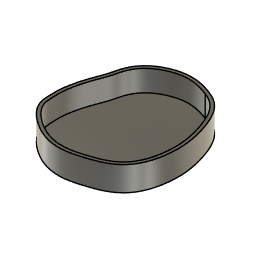
arm cover v3 (Autodesk Fusion 360 design; units mm, degrees)
Autodesk Fusion 360 part; units mm, degrees
sketch "Sketch1" plane through (0, 0, 0) normal (0, 0, 1) x (1, 0, 0)
  spline S0 degree 5 poles (4, 24) (4.2976, 23.8824) (4.8869, 23.6403) (5.7529, 23.2536) (6.872, 22.6708) (8.2119, 21.7595) (9.4914, 20.595) (10.706, 19.1267) (11.8468, 17.347) (12.9002, 15.3034) (13.8506, 13.0778) (14.6827, 10.7718) (15.3841, 8.4902) (15.9477, 6.3241) (16.3742, 4.3363) (16.6747, 2.5415) (16.8679, 0.9163) (16.9746, -0.5863) (17.014, -2.0239) (16.9985, -3.4508) (16.9299, -4.9045) (16.802, -6.407) (16.6033, -7.9648) (16.32, -9.5705) (15.9388, -11.2023) (15.4478, -12.8286) (14.8364, -14.413) (14.0949, -15.9199) (13.215, -17.3192) (12.1891, -18.5923) (11.0125, -19.7312) (9.6846, -20.7375) (8.2112, -21.6215) (6.6057, -22.4017) (4.8902, -23.1029) (3.0899, -23.7487) (1.2285, -24.3557) (-0.677, -24.9264) (-2.6203, -25.4435) (-4.6118, -25.8615) (-6.6717, -26.1171) (-8.8195, -26.1424) (-11.0657, -25.8772) (-13.4017, -25.2823) (-15.7921, -24.3507) (-18.162, -23.1234) (-20.4096, -21.6797) (-22.4258, -20.1182) (-24.1112, -18.5416) (-25.3954, -17.0399) (-26.253, -15.6745) (-26.7254, -14.4599) (-26.9274, -13.354) (-26.9931, -12.2827) (-27.0347, -11.1584) (-27.0876, -9.9025) (-27.1236, -8.4555) (-27.0862, -6.7846) (-26.9165, -4.8906) (-26.5879, -2.8189) (-26.1113, -0.6517) (-25.5211, 1.5133) (-24.867, 3.5786) (-24.2034, 5.467) (-23.5799, 7.1366) (-23.0304, 8.6046) (-22.5693, 9.9353) (-22.1911, 11.2109) (-21.8693, 12.5083) (-21.5539, 13.8703) (-21.1757, 15.2944) (-20.6627, 16.7519) (-19.9522, 18.1989) (-19.0061, 19.5914) (-17.8225, 20.8967) (-16.4248, 22.0905) (-14.8534, 23.154) (-13.1569, 24.0721) (-11.3826, 24.8303) (-9.5686, 25.413) (-7.7444, 25.8067) (-5.9328, 26.004) (-4.1503, 26.0067) (-2.409, 25.8296) (-0.7174, 25.505) (0.919, 25.0735) (2.1813, 24.6712) (3.1011, 24.3461) (3.7024, 24.1176) (4, 24) knots 0 0 0 0 0 0 0.01176471 0.02352941 0.03529412 0.04705882 0.05882353 0.07058824 0.08235294 0.09411765 0.10588235 0.11764706 0.12941176 0.14117647 0.15294118 0.16470588 0.17647059 0.18823529 0.2 0.21176471 0.22352941 0.23529412 0.24705882 0.25882353 0.27058824 0.28235294 0.29411765 0.30588235 0.31764706 0.32941176 0.34117647 0.35294118 0.36470588 0.37647059 0.38823529 0.4 0.41176471 0.42352941 0.43529412 0.44705882 0.45882353 0.47058824 0.48235294 0.49411765 0.50588235 0.51764706 0.52941176 0.54117647 0.55294118 0.56470588 0.57647059 0.58823529 0.6 0.61176471 0.62352941 0.63529412 0.64705882 0.65882353 0.67058824 0.68235294 0.69411765 0.70588235 0.71764706 0.72941176 0.74117647 0.75294118 0.76470588 0.77647059 0.78823529 0.8 0.81176471 0.82352941 0.83529412 0.84705882 0.85882353 0.87058824 0.88235294 0.89411765 0.90588235 0.91764706 0.92941176 0.94117647 0.95294118 0.96470588 0.97647059 0.98823529 1 1 1 1 1 1
  spline S1 degree 3 poles (4.9189, 26.325) (6.4748, 25.71) (8.0541, 24.968) (9.5874, 23.7829) (11.1792, 22.5526) (12.6425, 20.8269) (13.8702, 18.7373) (15.8899, 15.2997) (17.3679, 10.9247) (18.2619, 7.2921) (18.8769, 4.7933) (19.212, 2.6577) (19.3718, 0.7792) (19.5566, -1.3936) (19.5431, -3.2862) (19.3897, -5.3641) (19.2287, -7.5453) (18.8857, -9.9413) (18.1731, -12.396) (17.4873, -14.7578) (16.448, -17.1407) (14.8923, -19.1745) (13.489, -21.0092) (11.657, -22.5189) (9.6061, -23.6634) (7.6112, -24.7767) (5.446, -25.59) (3.2201, -26.3281) (1.1841, -27.0032) (-0.9009, -27.6409) (-3.2065, -28.1024) (-5.3968, -28.5409) (-7.8266, -28.7707) (-10.4262, -28.4313) (-13.0358, -28.0907) (-15.7974, -27.1537) (-18.3867, -25.7846) (-21.1672, -24.3144) (-23.7206, -22.4028) (-25.5919, -20.519) (-27.1445, -18.956) (-28.2367, -17.3891) (-28.8184, -15.8883) (-29.2502, -14.774) (-29.3878, -13.7475) (-29.4511, -12.9035) (-29.5261, -11.9028) (-29.5469, -11.0754) (-29.581, -9.9629) (-29.6197, -8.6986) (-29.6328, -7.0787) (-29.4342, -5.1952) (-29.1656, -2.6483) (-28.485, 0.3227) (-27.6743, 2.9569) (-27.0382, 5.024) (-26.3522, 6.8515) (-25.8115, 8.3076) (-25.2553, 9.8055) (-24.8726, 10.9085) (-24.557, 12.0964) (-24.2827, 13.1287) (-24.0484, 14.2937) (-23.6471, 15.6573) (-23.1884, 17.2158) (-22.4592, 18.9986) (-21.2879, 20.6179) (-19.7332, 22.7673) (-17.4837, 24.5713) (-15.0074, 25.8866) (-11.8886, 27.543) (-8.3863, 28.4728) (-5.0437, 28.482) (-2.733, 28.4883) (-0.5445, 28.0655) (1.4266, 27.5065) (2.6452, 27.1608) (3.7905, 26.771) (4.9189, 26.325) knots 0 0 0 0 0.03405552 0.03405552 0.03405552 0.06941006 0.06941006 0.06941006 0.12757193 0.12757193 0.12757193 0.16757966 0.16757966 0.16757966 0.21385419 0.21385419 0.21385419 0.2624294 0.2624294 0.2624294 0.30916723 0.30916723 0.30916723 0.35132881 0.35132881 0.35132881 0.39233682 0.39233682 0.39233682 0.42984722 0.42984722 0.42984722 0.46548177 0.46548177 0.46548177 0.50125441 0.50125441 0.50125441 0.53966828 0.53966828 0.53966828 0.5715399 0.5715399 0.5715399 0.59520385 0.59520385 0.59520385 0.62325635 0.62325635 0.62325635 0.65513731 0.65513731 0.65513731 0.69824515 0.69824515 0.69824515 0.73207311 0.73207311 0.73207311 0.76687413 0.76687413 0.76687413 0.79711827 0.79711827 0.79711827 0.83168571 0.83168571 0.83168571 0.87756774 0.87756774 0.87756774 0.9353539 0.9353539 0.9353539 0.97530131 0.97530131 0.97530131 1 1 1 1
  spline S2 degree 3 poles (5.4703, 27.72) (6.8981, 27.1557) (8.3804, 26.4768) (9.8776, 25.4307) (11.4843, 24.308) (13.0235, 22.7418) (14.3025, 20.8608) (16.2773, 17.9567) (17.7523, 14.3146) (18.8152, 10.8952) (19.5951, 8.3861) (20.1346, 6.0472) (20.4726, 4.017) (20.9323, 1.2555) (21.0378, -0.9634) (20.9931, -3.1848) (20.9542, -5.1171) (20.7976, -7.1205) (20.4174, -9.3083) (19.9666, -11.9023) (19.1978, -14.7226) (17.8111, -17.3661) (16.7276, -19.4316) (15.2256, -21.3659) (13.3818, -22.9008) (11.3936, -24.5559) (9.0775, -25.7248) (6.7476, -26.6495) (4.623, -27.4927) (2.4871, -28.1832) (0.1987, -28.8187) (-1.8091, -29.3762) (-3.9937, -29.8986) (-6.4754, -30.0538) (-8.8321, -30.2011) (-11.4382, -29.9579) (-14.0433, -29.1906) (-17.9011, -28.0542) (-21.7394, -25.8145) (-24.6953, -23.3621) (-26.5497, -21.8236) (-28.0514, -20.2274) (-29.108, -18.5854) (-29.9068, -17.3441) (-30.4328, -16.0283) (-30.6869, -14.8726) (-30.9062, -13.8755) (-30.9514, -13.0594) (-30.9866, -12.371) (-31.0292, -11.5369) (-31.0593, -10.7896) (-31.0866, -9.7902) (-31.1227, -8.4752) (-31.1206, -6.7466) (-30.8976, -4.7792) (-30.5937, -2.0973) (-29.8694, 0.9581) (-29.0376, 3.6251) (-28.3807, 5.7316) (-27.6846, 7.5697) (-27.1564, 8.995) (-26.6859, 10.2644) (-26.3612, 11.1981) (-26.0933, 12.1625) (-25.8477, 13.0466) (-25.6398, 14.0276) (-25.3126, 15.2666) (-24.9561, 16.6168) (-24.435, 18.2487) (-23.5374, 19.8695) (-22.5637, 21.6277) (-21.1605, 23.2993) (-19.52, 24.67) (-17.1742, 26.6301) (-14.4032, 28.0625) (-11.5186, 28.9633) (-8.9709, 29.7589) (-6.2911, 30.0928) (-3.7638, 29.9464) (-1.5974, 29.821) (0.4037, 29.3745) (2.2064, 28.8423) (3.3403, 28.5075) (4.405, 28.141) (5.4703, 27.72) knots 0 0 0 0 0.02986894 0.02986894 0.02986894 0.0619222 0.0619222 0.0619222 0.11141063 0.11141063 0.11141063 0.14772296 0.14772296 0.14772296 0.19711607 0.19711607 0.19711607 0.24008138 0.24008138 0.24008138 0.29102442 0.29102442 0.29102442 0.33083009 0.33083009 0.33083009 0.37375435 0.37375435 0.37375435 0.4128947 0.4128947 0.4128947 0.44723405 0.44723405 0.44723405 0.47984322 0.47984322 0.47984322 0.52813476 0.52813476 0.52813476 0.55842912 0.55842912 0.55842912 0.58133166 0.58133166 0.58133166 0.60109042 0.60109042 0.60109042 0.62502929 0.62502929 0.62502929 0.65652392 0.65652392 0.65652392 0.69945843 0.69945843 0.69945843 0.73337113 0.73337113 0.73337113 0.76357458 0.76357458 0.76357458 0.79126077 0.79126077 0.79126077 0.82142888 0.82142888 0.82142888 0.85415356 0.85415356 0.85415356 0.90095052 0.90095052 0.90095052 0.94228354 0.94228354 0.94228354 0.9777131 0.9777131 0.9777131 1 1 1 1
  point P0 (10.3723, 19.4695)
  point P1 (16, 6)
  point P2 (14, -16)
  point P3 (-1, -25)
  point P4 (-14, -25)
  point P5 (-26, -16)
  point P6 (-27, -12)
  point P7 (-27, -6)
  point P8 (-24, 6)
  point P9 (-22, 12)
  point P10 (-20, 18)
  point P11 (-13.2035, 24)
  point P12 (-3.8158, 25.9418)
  point P13 (17, -2)
  point P14 (16.5057, -8.4524)
  point P15 (8.5308, -21.3997)
  dimension "d1" = -2.5
  dimension "d2" = -4
extrude "Extrude1" add sketch "Sketch1" along normal blind 10 contours S2
extrude "Extrude2" add sketch "Sketch1" against normal blind 1.5 contours S0 | S1 | S2
equation "d2 = -2.5 mm - 1.5 mm"
named bodies: "left top arm connector-10mmheight"
